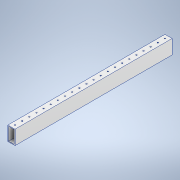
# Autodesk Inventor part: 22in2x1Extrusion
Saved by Autodesk Inventor 2020 (Build 240168000, 168)
## iProperties
Created: 2019-06-03
Part Number: 22in2x1Extrusion
Material: Aluminum 6061
Document SubType Name: Modeling
Designer: Connor
Density: 2.7 g/cm^3
Appearance: Aluminum - Flat
Author: Connor
Autodesk Inventor part; units mm, degrees
ref_plane "YZ Plane" through (0, 0, 0) normal (1, 0, 0) x (0, 1, 0)
ref_plane "XZ Plane" through (0, 0, 0) normal (0, 1, 0) x (-1, 0, 0)
ref_plane "XY Plane" through (0, 0, 0) normal (0, 0, 1) x (1, 0, 0)
sketch "Sketch1" plane through (0, 0, 0) normal (0, 0, 1) x (1, 0, 0)
  line L0 (0, 0) -> (25.4, 0)
  line L1 (25.4, 0) -> (25.4, 50.8)
  line L2 (25.4, 50.8) -> (0, 50.8)
  line L3 (0, 50.8) -> (0, 0)
  line L4 (2.54, 2.54) -> (22.86, 2.54)
  line L5 (22.86, 2.54) -> (22.86, 48.26)
  line L6 (22.86, 48.26) -> (2.54, 48.26)
  line L7 (2.54, 48.26) -> (2.54, 2.54)
  dimension "d0" = 25.4
  dimension "d1" = 50.8
  dimension "d2" = 2.54
  constraints: 16 end point, 4 parallel, 2 perpendicular, 1 horizontal, 3 other
  measures "d0" distance of L2.end L1.end
  measures "d1" distance of L1.end L0.end
  measures "d2" distance between parallel lines of L3 L7
extrude "Extrusion1" add sketch "Sketch1" along normal blind 558.8
sketch "Sketch2" plane through (0, 50.8, 0) normal (0, 1, 0) x (1, 0, 0)
  line L0 (25.4, -558.8) -> (0, -558.8) projected
  line L1 (0, 0) -> (0, -558.8) projected
  point P0 (12.7, -546.1)
  point P1 (12.7, -520.7)
  point P2 (12.7, -495.3)
  point P3 (12.7, -469.9)
  point P4 (12.7, -444.5)
  point P5 (12.7, -419.1)
  point P6 (12.7, -393.7)
  point P7 (12.7, -368.3)
  point P8 (12.7, -342.9)
  point P9 (12.7, -317.5)
  point P10 (12.7, -292.1)
  point P11 (12.7, -266.7)
  point P12 (12.7, -241.3)
  point P13 (12.7, -215.9)
  point P14 (12.7, -190.5)
  point P15 (12.7, -165.1)
  point P16 (12.7, -139.7)
  point P17 (12.7, -114.3)
  point P18 (12.7, -88.9)
  point P19 (12.7, -63.5)
  point P20 (12.7, -38.1)
  point P21 (12.7, -12.7)
  point P22 (12.7, 12.7)
  point P23 (12.7, 38.1)
  dimension "d5" = 12.7
  dimension "d6" = 12.7
  dimension "d9" = 25.4
  constraints: 1 vertical, 23 other
  measures "d5" distance from line of point (12.7, -546.1) L0
  measures "d6" distance from line of L1 point (12.7, -546.1)
  measures "d9" distance of point (12.7, -546.1) point (12.7, -520.7)
hole "Hole1" at (12.7, 50.8, 546.1) at (12.7, 50.8, 520.7) at (12.7, 50.8, 495.3) at (12.7, 50.8, 469.9) at (12.7, 50.8, 444.5) at (12.7, 50.8, 419.1) at (12.7, 50.8, 393.7) at (12.7, 50.8, 368.3) at (12.7, 50.8, 342.9) at (12.7, 50.8, 317.5) at (12.7, 50.8, 292.1) at (12.7, 50.8, 266.7) at (12.7, 50.8, 241.3) at (12.7, 50.8, 215.9) at (12.7, 50.8, 190.5) at (12.7, 50.8, 165.1) at (12.7, 50.8, 139.7) at (12.7, 50.8, 114.3) at (12.7, 50.8, 88.9) at (12.7, 50.8, 63.5) at (12.7, 50.8, 38.1) at (12.7, 50.8, 12.7) at (12.7, 50.8, -12.7) at (12.7, 50.8, -38.1) direction (0, -1, 0) diameter 4.1402 end through all
body "Solid1"
